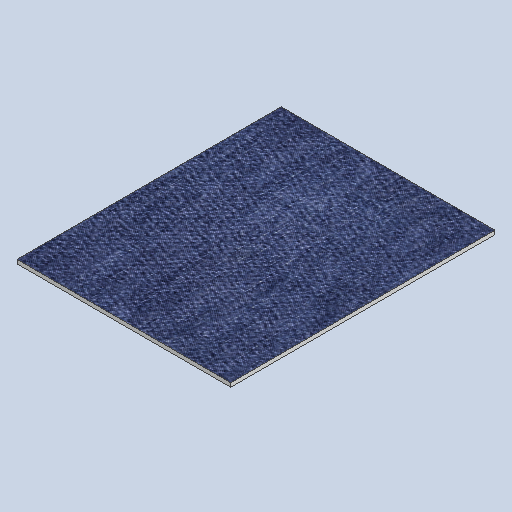
# Autodesk Inventor part: SolarPanel
Saved by Autodesk Inventor 2024.3 (Build 283343000, 343)
## iProperties
Created: 2025-01-15
Part Number: SolarPanel
Material: Generisch
Document SubType Name: Modeling
Designer: Maximilian Hock
Density: 1 g/cm^3
Appearance: Vorgabe
Author: Maximilian Hock
Autodesk Inventor part; units mm, degrees
ref_plane "YZ Plane" through (0, 0, 0) normal (1, 0, 0) x (0, 1, 0)
ref_plane "XZ Plane" through (0, 0, 0) normal (0, 1, 0) x (-1, 0, 0)
ref_plane "XY Plane" through (0, 0, 0) normal (0, 0, 1) x (1, 0, 0)
sketch "Skizze1" plane through (0, 0, 0) normal (0, 0, 1) x (1, 0, 0)
  line L0 (55, -68) -> (-55, -68)
  line L1 (-55, -68) -> (-55, 68)
  line L2 (-55, 68) -> (55, 68)
  line L3 (55, 68) -> (55, -68)
  line L4 (55, -68) -> (-55, 68) construction
  line L5 (-55, -68) -> (55, 68) construction
  point P0 (0, 0)
  dimension "d0" = 110
  dimension "d1" = 136
  constraints: 12 end point, 2 midpoint, 2 parallel, 1 horizontal, 1 perpendicular
  measures "d0" distance of L1.end L2.end
  measures "d1" distance of L0.end L1.end
extrude "Extrusion1" add sketch "Skizze1" along normal blind 2
sketch "Skizze2" plane through (0, 0, 0) normal (0, 0, 1) x (1, 0, 0)
  line L0 (-22.5, 23) -> (22.5, 23)
  line L1 (22.5, 23) -> (22.5, 60)
  line L2 (22.5, 60) -> (-22.5, 60)
  line L3 (-22.5, 60) -> (-22.5, 23)
  line L4 (-22.5, 23) -> (22.5, 60) construction
  line L5 (22.5, 23) -> (-22.5, 60) construction
  line L6 (55, 68) -> (-55, 68) projected
  line L7 (-3.5, 13) -> (3.5, 13)
  line L8 (3.5, 13) -> (3.5, 23)
  line L9 (3.5, 23) -> (-3.5, 23)
  line L10 (-3.5, 23) -> (-3.5, 13)
  line L11 (-3.5, 13) -> (3.5, 23) construction
  line L12 (3.5, 13) -> (-3.5, 23) construction
  point P0 (0, 0)
  point P1 (0, 41.5)
  point P2 (0, 18)
  dimension "d4" = 45
  dimension "d5" = 37
  dimension "d6" = 8
  dimension "d7" = 7
  dimension "d8" = 10
  constraints: 24 end point, 4 midpoint, 4 parallel, 2 horizontal, 2 perpendicular, 2 vertical alignment, 1 point on line
  measures "d4" distance of L1.end L2.end
  measures "d5" distance of L0.end L1.end
  measures "d6" distance between parallel lines of L6 L2
  measures "d7" distance of L7.start L7.end
  measures "d8" distance of L7.end L8.end
extrude "Extrusion2" add sketch "Skizze2" against normal blind 8
equation "\"d0\" = SolarPanelWidth"
equation "\"d1\" = SolarPanelHeight"
equation "\"d2\" = SolarPanelThickness"
equation "\"d4\" = SolarPanelConnectorWidth"
equation "\"d5\" = SolarPanelConnectorHeight"
equation "\"d9\" = SolarPanelConnectorDepth"
equation "\"SolarPanelWidth\" = 110"
equation "\"SolarPanelHeight\" = 136"
equation "\"SolarPanelThickness\" = 2"
equation "\"SolarPanelConnectorWidth\" = 45"
equation "\"SolarPanelConnectorHeight\" = 37"
equation "\"SolarPanelConnectorDepth\" = 8"
